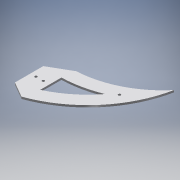
# Autodesk Inventor part: landing-gear-claws
Saved by Autodesk Inventor 2016 (Build 200138000, 138)
## iProperties
Created: 2015-01-28
Part Number: landing-gear-claws
Material: ABS Plastic
Document SubType Name: Modeling
Designer: Vasanth
Density: 1.06 g/cm^3
Appearance: Smooth - White
Mass: 4.49481 g
Surface Area: 51.5481 cm^2
Volume: 4.24039 cm^3
Author: Vasanth
Autodesk Inventor part; units mm, degrees
ref_plane "YZ Plane" through (0, 0, 0) normal (1, 0, 0) x (0, 1, 0)
ref_plane "XZ Plane" through (0, 0, 0) normal (0, 1, 0) x (-1, 0, 0)
ref_plane "XY Plane" through (0, 0, 0) normal (0, 0, 1) x (1, 0, 0)
sketch "Sketch12" plane through (0, 0, 0) normal (0, 1, 0) x (-1, 0, 0)
  arc A0 (-17.9101, 19.3197) -> (-99.957, -10.5429) centre (-33.0718, -66.6663) ccw
  arc A1 (-36.0097, 32.8266) -> (-70.4306, 25.593) centre (-33.0718, -66.6663) ccw
  circle A2 centre (-30.1338, 44.1595) radius 1.016
  line L0 (-36.0097, 32.8266) -> (-36.0097, 53.0201)
  arc A3 (-36.0097, 53.0201) -> (-70.4306, 25.593) centre (2.8014, -31.0003) ccw
  line L1 (-17.9101, 19.3197) -> (-17.9101, 71.7072)
  arc A4 (-17.9101, 71.7072) -> (-99.957, -10.5429) centre (2.8014, -31.0003) ccw
  circle A5 centre (-30.1338, 44.1595) radius 1.2065
  circle A6 centre (-77.8759, 19.3514) radius 1.2065
  constraints: 8 point on circle, 7 centre point, 4 end point, 2 vertical, 1 coincident
extrude "Extrusion13" add sketch "Sketch12" along normal blind 1.905 contours A0 A4 L1
sketch "Sketch20" plane through (0, 1.905, 0) normal (0, 1, 0) x (1, 0, 0)
  circle A0 centre (30.1338, -44.1595) radius 1.2065 projected
  line L0 (30.1338, -42.953) -> (30.1338, -44.1595)
  line L1 (30.1338, -44.1595) -> (23.098, -44.1595)
  circle A1 centre (23.098, -44.1595) radius 1.2065
  point P0 (0, 0)
  dimension "d94" = 7.0358
  constraints: 4 end point, 1 centre point, 1 coincident, 1 perpendicular, 1 vertical, 1 vertical alignment, 1 other
  measures "d94" distance of L0.end L1.end
extrude "Extrusion15" cut sketch "Sketch20" against normal blind 3.175 contours A1
sketch "Sketch22" plane through (0, 1.905, 0) normal (0, 1, 0) x (1, 0, 0)
  line L0 (17.9101, -19.3197) -> (17.9101, -71.7072) projected
  line L1 (17.9101, -19.3197) -> (17.9101, -32.0197)
  line L2 (17.9101, -32.0197) -> (37.8348, -20.5162)
  arc A0 (17.9101, -71.7072) -> (99.957, 10.5429) centre (-2.8014, 31.0003) ccw projected
  line L3 (17.9101, -71.7072) -> (17.9101, -59.0072)
  line L4 (17.9101, -59.0072) -> (32.7327, -67.565)
  arc A1 (17.9101, -71.7072) -> (32.7327, -67.565) centre (-2.8014, 31.0003) ccw
  arc A2 (17.9101, -19.3197) -> (99.957, 10.5429) centre (33.0718, 66.6663) ccw projected
  arc A3 (17.9101, -19.3197) -> (37.8348, -20.5162) centre (33.0718, 66.6663) ccw
  point P0 (0, 0)
  dimension "d103" = 12.7
  dimension "d104" = 60
  dimension "d105" = 12.7
  dimension "d106" = 60
  constraints: 8 end point, 4 point on circle, 4 point on line, 2 centre point, 2 coincident, 1 concentric
  measures "d103" distance of L0.start L1.end
  measures "d104" angle of L2 L1
  measures "d105" distance of L0.end L3.end
  measures "d106" angle of L3 L4
extrude "Extrusion17" cut sketch "Sketch22" against normal blind 3.175 contours A2 L2 L0 | L4 A0 L0
move or copy body "Move Body1" bodies to move or copy 1 copy no rotation origin (0, 0, 0) rotation axis (0, 0, 1) rotation angle -90 translate (16.0051, 19.8151, 0)
move or copy body "Move Body2" bodies to move or copy 1 copy no rotation origin (0, 0, 0) rotation axis (0, 0, 1) rotation angle 90 translate (19.8151, -16.0051, 0)
body "Solid2"
